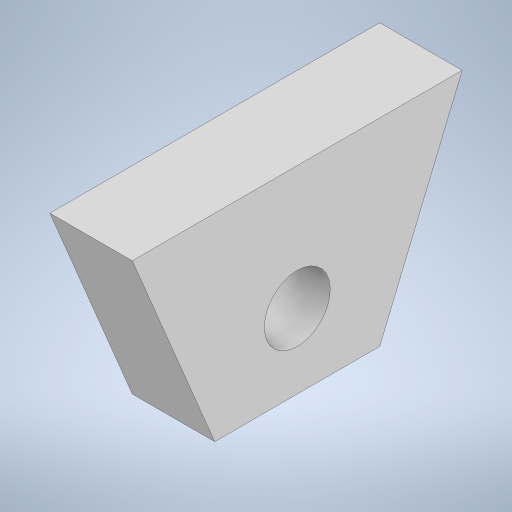
# Autodesk Inventor part: task2
Saved by Autodesk Inventor 2024.2 (Build 282272000, 272)
## iProperties
Created: 2024-10-18
Part Number: task2
Material: Типовые
Document SubType Name: Modeling
Designer: user
Density: 1 g/cm^3
Appearance: По умолчанию
Author: user
Autodesk Inventor part; units mm, degrees
ref_plane "YZ Plane" through (0, 0, 0) normal (1, 0, 0) x (0, 1, 0)
ref_plane "XZ Plane" through (0, 0, 0) normal (0, 1, 0) x (-1, 0, 0)
ref_plane "XY Plane" through (0, 0, 0) normal (0, 0, 1) x (1, 0, 0)
sketch "Эскиз1" plane through (0, 0, 0) normal (1, 0, 0) x (0, 1, 0)
  line L0 (0, 0) -> (0, -10)
  line L1 (0, -10) -> (0, 10)
  line L2 (24, 0) -> (24, -20)
  line L3 (24, -20) -> (24, 20)
  line L4 (0, 10) -> (24, 20)
  line L5 (0, -10) -> (24, -20)
  circle A0 centre (9, 0) radius 4
  constraints: 12 end point, 3 vertical, 1 centre point, 1 point on line
extrude "Выдавливание1" add sketch "Эскиз1" along normal blind 10
